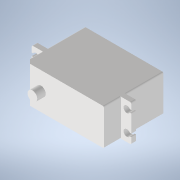
# Autodesk Inventor part: Servo
Saved by Autodesk Inventor 2020.3 (Build 243373010, 373A)
## iProperties
Created: 2020-12-08
Part Number: Servo
Material: Generisch
Document SubType Name: Modeling
Designer: Stefan
Density: 1 g/cm^3
Appearance: Vorgabe
Author: Stefan
Autodesk Inventor part; units mm, degrees
ref_plane "YZ Plane" through (0, 0, 0) normal (1, 0, 0) x (0, 1, 0)
ref_plane "XZ Plane" through (0, 0, 0) normal (0, 1, 0) x (-1, 0, 0)
ref_plane "XY Plane" through (0, 0, 0) normal (0, 0, 1) x (1, 0, 0)
sketch "Skizze1" plane through (0, 0, 0) normal (0, 0, 1) x (1, 0, 0)
  line L0 (-12, 15) -> (51, 15)
  line L1 (52, 14) -> (52, -14)
  line L2 (51, -15) -> (-12, -15)
  line L3 (-13, -14) -> (-13, 14)
  arc A0 (-12, 15) -> (-13, 14) centre (-12, 14) ccw
  arc A1 (-13, -14) -> (-12, -15) centre (-12, -14) ccw
  arc A2 (51, -15) -> (52, -14) centre (51, -14) ccw
  arc A3 (52, 14) -> (51, 15) centre (51, 14) ccw
  point P0 (0, 0)
  point P1 (-13, 15)
  point P2 (52, 15)
  point P3 (-13, -15)
  dimension "d0" = 65
  dimension "d1" = 30
  dimension "d2" = 15
  dimension "d3" = 13
  dimension "d4" = 1
  constraints: 8 end point, 8 point on circle, 8 tangent, 6 point on line, 4 centre point, 3 equal radius, 2 parallel, 1 horizontal, 1 perpendicular
  measures "d0" distance of point (-13, 15) point (52, 15)
  measures "d1" distance of point (-13, -15) point (-13, 15)
  measures "d2" distance from line of L0 point (0, 0)
  measures "d3" distance from line of point (0, 0) L3
  measures "d4" radius of A0
extrude "Extrusion1" add sketch "Skizze1" along normal blind 31
sketch "Skizze2" plane through (0, 0, 31) normal (0, 0, 1) x (1, 0, 0)
  line L0 (-20.5, 15) -> (59.5, 15)
  line L1 (59.5, -15) -> (-20.5, -15)
  arc A0 (-20.5, 15) -> (-21.5, 14) centre (-20.5, 14) ccw
  arc A1 (-21.5, -14) -> (-20.5, -15) centre (-20.5, -14) ccw
  arc A2 (59.5, -15) -> (60.5, -14) centre (59.5, -14) ccw
  arc A3 (60.5, 14) -> (59.5, 15) centre (59.5, 14) ccw
  arc A4 (-20.3995, 7.2) -> (-20.3995, 9.7) centre (-17.95, 8.45) ccw
  arc A5 (-20.3995, -9.7) -> (-20.3995, -7.2) centre (-17.95, -8.45) ccw
  line L2 (-20.3995, -7.2) -> (-21.5, -7.2)
  line L3 (-21.5, -9.7) -> (-20.3995, -9.7)
  line L4 (-21.5, -14) -> (-21.5, -9.7)
  line L5 (-20.3995, 9.7) -> (-21.5, 9.7)
  line L6 (-21.5, 7.2) -> (-20.3995, 7.2)
  line L7 (-21.5, -7.2) -> (-21.5, 7.2)
  line L8 (-21.5, 9.7) -> (-21.5, 14)
  line L9 (19.5, 16.9478) -> (19.5, -22.1923) construction
  arc A6 (59.3995, 9.7) -> (59.3995, 7.2) centre (56.95, 8.45) ccw
  arc A7 (59.3995, -7.2) -> (59.3995, -9.7) centre (56.95, -8.45) ccw
  line L10 (59.3995, -7.2) -> (60.5, -7.2)
  line L11 (60.5, -9.7) -> (59.3995, -9.7)
  line L12 (60.5, -14) -> (60.5, -9.7)
  line L13 (59.3995, 9.7) -> (60.5, 9.7)
  line L14 (60.5, 7.2) -> (59.3995, 7.2)
  line L15 (60.5, -7.2) -> (60.5, 7.2)
  line L16 (60.5, 9.7) -> (60.5, 14)
  point P0 (0, 0)
  point P1 (60.5, -15)
  point P2 (60.5, 15)
  dimension "d7" = 30
  dimension "d10" = 1
  dimension "d11" = 15
  dimension "d12" = 5.5
  dimension "d13" = 5.5
  dimension "d14" = 6.55
  dimension "d15" = 6.55
  dimension "d19" = 1.25
  dimension "d23" = 1.25
  dimension "d25" = 41
  dimension "d26" = 21.5
  constraints: 34 end point, 16 point on circle, 10 symmetric about line, 10 tangent, 8 centre point, 3 equal radius, 3 horizontal, 3 parallel, 2 point on line, 2 other
  measures "d7" distance of point (60.5, 15) point (60.5, -15)
  measures "d10" radius of A0
  measures "d11" distance from line of L0 point (0, 0)
  measures "d12" diameter of A4
  measures "d13" diameter of A5
  measures "d14" distance from line of L0 A4.centre
  measures "d15" distance from line of A5.centre L1
  measures "d19" distance from line of L2 A5.centre
  measures "d23" distance from line of A4.centre L5
  measures "d25" distance between parallel lines of L7 L9
  measures "d26" distance from line of L7 point (0, 0)
extrude "Extrusion2" add sketch "Skizze2" along normal blind 4
sketch "Skizze3" plane through (0, 0, 35) normal (0, 0, 1) x (1, 0, 0)
  line L0 (-12, 15) -> (51, 15)
  line L1 (52, 14) -> (52, -14)
  line L2 (51, -15) -> (-12, -15)
  line L3 (-13, -14) -> (-13, 14)
  arc A0 (-12, 15) -> (-13, 14) centre (-12, 14) ccw
  arc A1 (-13, -14) -> (-12, -15) centre (-12, -14) ccw
  arc A2 (51, -15) -> (52, -14) centre (51, -14) ccw
  arc A3 (52, 14) -> (51, 15) centre (51, 14) ccw
  point P0 (0, 0)
  point P1 (0, 0)
  point P2 (-13, 15)
  point P3 (52, 15)
  point P4 (-13, -15)
  dimension "d29" = 65
  dimension "d30" = 30
  dimension "d31" = 15
  dimension "d32" = 13
  dimension "d33" = 1
  constraints: 8 end point, 8 point on circle, 8 tangent, 6 point on line, 4 centre point, 3 equal radius, 2 parallel, 1 horizontal, 1 perpendicular
  measures "d29" distance of point (-13, 15) point (52, 15)
  measures "d30" distance of point (-13, -15) point (-13, 15)
  measures "d31" distance from line of L0 point (0, 0)
  measures "d32" distance from line of point (0, 0) L3
  measures "d33" radius of A0
extrude "Extrusion3" add sketch "Skizze3" along normal blind 14
chamfer "Fase1" distance 4 angle 45 1 edges at (-13, 0, 49)
sketch "Skizze4" plane through (0, 0, 49) normal (0, 0, 1) x (1, 0, 0)
  circle A0 centre (0, 0) radius 4
  dimension "d39" = 8
  constraints: 1 centre point, 1 coincident
  measures "d39" diameter of A0
extrude "Extrusion4" add sketch "Skizze4" along normal blind 7
